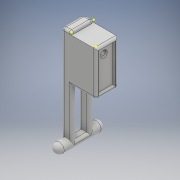
# Autodesk Inventor part: bal
Saved by Autodesk Inventor 2018 (Build 220112000, 112)
## iProperties
Created: 2019-11-11
Part Number: bal
Material: 일반
Document SubType Name: Modeling
Designer: LeeYounSeo
Density: 1 g/cm^3
Appearance: 기본값
Author: LeeYounSeo
Autodesk Inventor part; units mm, degrees
ref_plane "YZ Plane" through (0, 0, 0) normal (1, 0, 0) x (0, 1, 0)
ref_plane "XZ Plane" through (0, 0, 0) normal (0, 1, 0) x (-1, 0, 0)
ref_plane "XY Plane" through (0, 0, 0) normal (0, 0, 1) x (1, 0, 0)
sketch "스케치1" plane through (0, 0, 0) normal (0, 1, 0) x (-1, 0, 0)
  line L0 (0, 0) -> (4, 0)
  line L1 (4, 0) -> (4, -40)
  line L2 (4, -40) -> (0, -40)
  line L3 (0, -40) -> (0, 0)
  dimension "d0" = 40
  dimension "d1" = 4
  constraints: 8 end point, 2 parallel, 1 horizontal, 1 perpendicular
  measures "d0" distance of L0.end L1.end
  measures "d1" distance of L1.end L2.end
extrude "돌출1" add sketch "스케치1" along normal blind 9
sketch "스케치3" plane through (0, 9, 0) normal (0, 1, 0) x (1, 0, 0)
  line L0 (0, 40) -> (-4, 40) projected
  circle A0 centre (-2, 40) radius 2
  point P0 (0, 0)
  constraints: 1 horizontal alignment, 1 midpoint, 2 other
extrude "돌출3" add sketch "스케치3" along normal mid plane 10
sketch "스케치4" plane through (0, 0, 0) normal (0, -1, 0) x (1, 0, 0)
  point P0 (0, 0)
sketch "스케치5" plane through (0, 0, 0) normal (0, -1, 0) x (1, 0, 0)
  line L0 (-4, -40) -> (0, -40) projected
  circle A0 centre (-2, -40) radius 2
  point P0 (0, 0)
  constraints: 1 horizontal alignment, 1 midpoint, 2 other
extrude "돌출4" add sketch "스케치5" along normal mid plane 10
fillet "모깎기1" radius 2 2 edges at (-4, 14, -40) (-4, -5, -40)
sketch "스케치6" plane through (0, 0, 0) normal (1, 0, 0) x (0, 0, -1)
  line L0 (39, 7) -> (19.9, 7)
  line L1 (19.9, 7) -> (19.9, 2)
  line L2 (19.9, 2) -> (39, 2)
  line L3 (39, 2) -> (39, 7)
  line L4 (40, 0) -> (0, 0) projected
  line L5 (0, 9) -> (40, 9) projected
  line L6 (16.9, 7.8) -> (16.9, 1) projected
  line L7 (40, 0) -> (40, 9) projected
  dimension "d15" = 2
  dimension "d16" = 2
  dimension "d17" = 3
  dimension "d18" = 1
  constraints: 8 end point, 2 parallel, 1 horizontal, 1 perpendicular
  measures "d15" distance between parallel lines of L4 L2
  measures "d16" distance between parallel lines of L5 L0
  measures "d17" distance between parallel lines of L6 L1
  measures "d18" distance between parallel lines of L7 L3
extrude "돌출5" cut sketch "스케치6" against normal blind 10
fillet "모깎기2" radius 1 6 edges at (-2, 9, 0) (0, 4.5, 0) (-2, 0, 0) (-4, 4.5, 0) (0, 0, -20) (-4, 0, -20)
fillet "모깎기3" radius 1 4 edges at (-0.2929, 8.7071, -0.2929) (0, 9, -20.5) (-3.7071, 8.7071, -0.2929) (-4, 9, -20.5)
fillet "모깎기4" radius 1 5 edges at (0, 4.5, -39) (-4, 4.5, -39) (0, 2, -29.45) (0, 7, -29.45) (0, 4.5, -19.9)
fillet "모깎기5" radius 1 5 edges at (-4, 2, -39.4999) (-4, 2, -29.45) (-4, 4.5, -19.9) (-4, 7, -39.4999) (-4, 7, -29.45)
sketch "스케치9" plane through (0, 1, -1) normal (1, 0, 0) x (0, 0, -1)
  line L0 (17.9, 7) -> (17.9, 0) projected
  line L1 (0, 7) -> (17.9, 7) projected
  line L2 (0, 0) -> (0, 7) projected
  line L3 (17.9, 0) -> (0, 0) projected
  point P0 (-1, -1)
extrude "돌출7" add sketch "스케치9" along normal blind 10
sketch "스케치10" plane through (10, 1, -1) normal (1, 0, 0) x (0, 0, -1)
  point P0 (-1, -1)
sketch "스케치11" plane through (-4, 1, -1) normal (-1, 0, 0) x (0, 0, 1)
  line L0 (-1, 6.9) -> (-17, 6.9)
  line L1 (-17, 6.9) -> (-17, 0.1)
  line L2 (-17, 0.1) -> (-1, 0.1)
  line L3 (-1, 0.1) -> (-1, 6.9)
  line L4 (0, 0) -> (-17.9, 0) projected
  line L5 (0, 7) -> (0, 0) projected
  point P0 (1, -1)
  dimension "d36" = 16
  dimension "d37" = 6.8
  dimension "d38" = 0.1
  dimension "d39" = 1
  constraints: 8 end point, 2 parallel, 1 horizontal, 1 perpendicular
  measures "d36" distance of L1.end L2.end
  measures "d37" distance of L2.end L0.start
  measures "d38" distance between parallel lines of L2 L4
  measures "d39" distance between parallel lines of L3 L5
extrude "돌출8" cut sketch "스케치11" against normal blind 11.5
sketch "스케치12" plane through (10, 1, -1) normal (1, 0, 0) x (0, 0, -1)
  line L0 (0.9, 6.9) -> (16.9, 6.9)
  line L1 (16.9, 6.9) -> (16.9, 0.1)
  line L2 (16.9, 0.1) -> (0.9, 0.1)
  line L3 (0.9, 0.1) -> (0.9, 6.9)
  line L4 (17.9, 0) -> (17.9, 7) projected
  line L5 (0, 0) -> (17.9, 0) projected
  point P0 (-1, -1)
  dimension "d42" = 16
  dimension "d43" = 6.8
  dimension "d44" = 1
  dimension "d45" = 0.1
  constraints: 8 end point, 2 parallel, 1 horizontal, 1 perpendicular
  measures "d42" distance of L1.end L2.end
  measures "d43" distance of L2.end L0.start
  measures "d44" distance between parallel lines of L4 L1
  measures "d45" distance between parallel lines of L5 L2
extrude "돌출9" cut sketch "스케치12" against normal blind 1.3
sketch "스케치13" plane through (0, 1, -18.9) normal (0, -1, 0) x (1, 0, 0)
  line L0 (0, 0) -> (0, 17.9) projected
  line L1 (0, 0) -> (10, 0) projected
  line L2 (10, 17.9) -> (10, 0) projected
  line L3 (0, 17.9) -> (10, 17.9) projected
  point P0 (0, 18.9)
extrude "돌출10" add sketch "스케치13" along normal blind 1
sketch "스케치14" plane through (0, 8, -1) normal (0, 1, 0) x (1, 0, 0)
  line L0 (0, 0) -> (0, 17.9) projected
  line L1 (0, 0) -> (10, 0) projected
  line L2 (10, 17.9) -> (10, 0) projected
  line L3 (0, 17.9) -> (10, 17.9) projected
  point P0 (0, -1)
extrude "돌출11" add sketch "스케치14" along normal blind 1
sketch "스케치15" plane through (10, 1, -1) normal (1, 0, 0) x (0, 0, -1)
  line L0 (0.9, 0.1) -> (0.9, 6.9) projected
  line L1 (0.9, 6.9) -> (16.9, 6.9) projected
  line L2 (16.9, 6.9) -> (16.9, 0.1) projected
  line L3 (16.9, 0.1) -> (0.9, 0.1) projected
  line L4 (17.9, 8) -> (17.9, -1) projected
  line L5 (0, 8) -> (17.9, 8) projected
  line L6 (0, -1) -> (0, 8) projected
  line L7 (17.9, -1) -> (0, -1) projected
  point P0 (-1, -1)
extrude "돌출12" add sketch "스케치15" against normal blind 11
sketch "스케치16" plane through (8.7, 1, -1) normal (1, 0, 0) x (0, 0, -1)
  circle A0 centre (4.4, 3.4) radius 1.4
  line L0 (0.9, 0.1) -> (0.9, 6.9) projected
  line L1 (0.9, 6.9) -> (16.9, 6.9) projected
  point P0 (-1, -1)
  dimension "d54" = 2.8
  dimension "d55" = 3.5
  dimension "d56" = 3.5
  constraints: 1 centre point
  measures "d54" diameter of A0
  measures "d55" distance from line of A0.centre L0
  measures "d56" distance from line of L1 A0.centre
extrude "돌출13" cut sketch "스케치16" against normal blind 11
sketch "스케치17" plane through (7.5, 1, -1) normal (-1, 0, 0) x (0, 0, 1)
  circle A0 centre (-4.4, 3.4) radius 2.4
  circle A1 centre (-4.4, 3.4) radius 1.4 projected
  point P0 (1, -1)
  dimension "d59" = 4.8
  dimension "d60" = 0
  dimension "d61" = 0
  constraints: 1 centre point
  measures "d59" diameter of A0
  measures "d60" distance of A1.centre A0.centre
  measures "d61" distance of A0.centre A1.centre
extrude "돌출14" cut sketch "스케치17" against normal blind 0.5
fillet "모깎기6" radius 1 6 edges at (10, 4.5, -1) (10, 0, -9.95) (10, 9, -9.95) (10, 4.5, -18.9) (4.5, 0, -18.9) (4.5, 9, -18.9)
sketch "스케치19" plane through (-4, 1, -1) normal (-1, 0, 0) x (0, 0, 1)
  line L0 (-17.9, 7) -> (0, 7) projected
  line L1 (0, 0) -> (-17.9, 0) projected
  line L2 (-17.9, 7) -> (-7.7404, 7)
  line L3 (-7.7404, 7) -> (-7.7404, 0)
  line L4 (-7.7404, 0) -> (-17.9, 0)
  line L5 (-17.9, 0) -> (-17.9, 7)
  point P0 (1, -1)
  constraints: 8 end point, 2 parallel, 1 horizontal, 1 perpendicular, 1 point on line
extrude "돌출16" add sketch "스케치19" against normal blind 11.4
fillet "모깎기7" radius 1 8 edges at (-2.5, 7.9, -2) (3.25, 7.9, -2) (-2.5, 1.1, -2) (3.25, 1.1, -2) (-2.5, 7.9, -8.7404) (3.2, 7.9, -8.7404) (-2.5, 1.1, -8.7404) (3.2, 1.1, -8.7404)
sketch "스케치20" plane through (0, 9, 0) normal (0, 1, 0) x (1, 0, 0)
  point P0 (0, 0)
